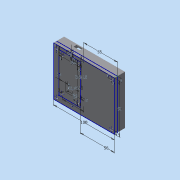
# Autodesk Inventor part: Base_V1
Saved by Autodesk Inventor 2015 (Build 190159000, 159)
## iProperties
Created: 2014-12-24
Part Number: Base_V1
Material: Generic
Document SubType Name: Modeling
Designer: Openlab
Density: 1 g/cm^3
Appearance: Default
Author: Openlab
Autodesk Inventor part; units mm, degrees
ref_plane "YZ Plane" through (0, 0, 0) normal (1, 0, 0) x (0, 1, 0)
ref_plane "XZ Plane" through (0, 0, 0) normal (0, 1, 0) x (-1, 0, 0)
ref_plane "XY Plane" through (0, 0, 0) normal (0, 0, 1) x (1, 0, 0)
sketch "Sketch1" plane through (0, 0, 0) normal (0, 1, 0) x (-1, 0, 0)
  line L0 (100, 0) -> (0, 0)
  line L1 (0, 0) -> (0, -80)
  line L2 (0, -80) -> (100, -80)
  line L3 (100, -80) -> (100, 0)
  line L4 (95, -5) -> (78, -5)
  line L5 (5, -5) -> (5, -75)
  line L6 (5, -75) -> (95, -75)
  line L7 (95, -75) -> (95, -5)
  line L8 (33.5, -10) -> (23.5, -10)
  line L9 (23.5, -10) -> (23.5, -20)
  line L10 (23.5, -20) -> (33.5, -20)
  line L11 (95, -65) -> (95, -5)
  line L12 (33.5, -50) -> (23.5, -50)
  line L13 (23.5, -50) -> (23.5, -60)
  line L14 (23.5, -60) -> (33.5, -60)
  line L15 (95, -5) -> (90, -5)
  line L16 (90, -5) -> (90, -10)
  line L17 (90, -10) -> (95, -10)
  line L18 (95, -10) -> (95, -5)
  line L19 (95, -75) -> (90, -75)
  line L20 (90, -75) -> (90, -70)
  line L21 (90, -70) -> (95, -70)
  line L22 (95, -70) -> (95, -75)
  line L23 (5, -5) -> (10, -5)
  line L24 (10, -5) -> (10, -10)
  line L25 (10, -10) -> (5, -10)
  line L26 (5, -10) -> (5, -5)
  line L27 (5, -75) -> (10, -75)
  line L28 (10, -75) -> (10, -70)
  line L29 (10, -70) -> (5, -70)
  line L30 (5, -70) -> (5, -75)
  line L31 (78, -5) -> (78, -2.5)
  line L32 (78, -2.5) -> (68, -2.5)
  line L33 (68, -2.5) -> (68, -5)
  line L34 (78, -5) -> (73, -5) construction
  line L35 (95, -5) -> (78, -5)
  line L36 (73, -5) -> (68, -5) construction
  line L37 (68, -5) -> (55, -5)
  line L38 (14.5, -63) -> (14.5, -5)
  line L39 (38.5, -63) -> (14.5, -63)
  line L40 (14.5, -5) -> (5, -5)
  line L41 (33.5, -30) -> (23.5, -30)
  line L42 (23.5, -30) -> (23.5, -40)
  line L43 (23.5, -40) -> (33.5, -40)
  line L44 (35.5, -60) -> (36.6, -60)
  line L45 (36.6, -50) -> (35.5, -50)
  line L46 (33.5, -60) -> (33.5, -56.5)
  line L47 (33.5, -53.5) -> (33.5, -50)
  line L48 (38.5, -56.5) -> (38.5, -63)
  line L49 (36.6, -60) -> (36.6, -56.5)
  line L50 (36.6, -53.5) -> (36.6, -50)
  line L51 (35.5, -50) -> (35.5, -53.5)
  line L52 (35.5, -56.5) -> (35.5, -60)
  line L53 (33.5, -56.5) -> (35.5, -56.5)
  line L54 (36.6, -56.5) -> (38.5, -56.5)
  line L55 (38.5, -53.5) -> (36.6, -53.5)
  line L56 (35.5, -53.5) -> (33.5, -53.5)
  line L57 (33.5, -40) -> (33.5, -36.5)
  line L58 (33.5, -33.5) -> (33.5, -30)
  line L59 (38.5, -36.5) -> (38.5, -53.5)
  line L60 (33.5, -20) -> (33.5, -16.5)
  line L61 (33.5, -13.5) -> (33.5, -10)
  line L62 (38.5, -5) -> (38.5, -13.5)
  line L63 (38.5, -16.5) -> (38.5, -33.5)
  line L64 (35.5, -40) -> (36.6, -40)
  line L65 (36.6, -30) -> (35.5, -30)
  line L66 (38.5, -36.5) -> (36.6, -36.5)
  line L67 (35.5, -36.5) -> (33.5, -36.5)
  line L68 (38.5, -33.5) -> (36.6, -33.5)
  line L69 (35.5, -33.5) -> (33.5, -33.5)
  line L70 (35.5, -30) -> (35.5, -33.5)
  line L71 (35.5, -36.5) -> (35.5, -40)
  line L72 (36.6, -40) -> (36.6, -36.5)
  line L73 (36.6, -33.5) -> (36.6, -30)
  line L74 (35.5, -20) -> (36.6, -20)
  line L75 (36.6, -10) -> (35.5, -10)
  line L76 (33.5, -16.5) -> (35.5, -16.5)
  line L77 (36.6, -16.5) -> (38.5, -16.5)
  line L78 (33.5, -13.5) -> (35.5, -13.5)
  line L79 (36.6, -13.5) -> (38.5, -13.5)
  line L80 (35.5, -10) -> (35.5, -13.5)
  line L81 (35.5, -16.5) -> (35.5, -20)
  line L82 (36.6, -20) -> (36.6, -16.5)
  line L83 (36.6, -13.5) -> (36.6, -10)
  line L84 (33.5, -56.5) -> (33.5, -53.5)
  line L85 (38.5, -56.5) -> (38.5, -53.5)
  line L86 (38.5, -36.5) -> (38.5, -33.5)
  line L87 (33.5, -36.5) -> (33.5, -33.5)
  line L88 (33.5, -16.5) -> (33.5, -13.5)
  line L89 (38.5, -16.5) -> (38.5, -13.5)
  line L90 (14.5, -57.5) -> (23.5, -57.5)
  line L91 (14.5, -52.5) -> (23.5, -52.5)
  line L92 (14.5, -37.5) -> (23.5, -37.5)
  line L93 (14.5, -32.5) -> (23.5, -32.5)
  line L94 (14.5, -17.5) -> (23.5, -17.5)
  line L95 (14.5, -12.5) -> (23.5, -12.5)
  line L96 (35.5, -56.5) -> (35.5, -53.5)
  line L97 (36.6, -56.5) -> (36.6, -53.5)
  line L98 (35.5, -36.5) -> (35.5, -33.5)
  line L99 (36.6, -36.5) -> (36.6, -33.5)
  line L100 (35.5, -16.5) -> (35.5, -13.5)
  line L101 (36.6, -16.5) -> (36.6, -13.5)
  line L102 (40, -5) -> (40, -63)
  line L103 (68, -5) -> (43, -5)
  line L104 (40, -5) -> (38.5, -5)
  line L105 (37, -75) -> (37, -72)
  line L106 (40, -5) -> (43, -5)
  line L107 (13, -5) -> (13, -72)
  line L108 (13, -72) -> (14.5, -72)
  line L109 (10, -71) -> (10, -5)
  line L110 (14.5, -72) -> (14.5, -75)
  line L111 (2.5002, -77.5) -> (2.5002, -2.5)
  line L112 (2.5002, -2.5) -> (97.5, -2.5)
  line L113 (97.5, -2.5) -> (97.5, -77.5)
  line L114 (97.5, -77.5) -> (2.5002, -77.5)
  line L115 (40, -63) -> (43, -63)
  line L116 (43, -75) -> (43, -72)
  line L117 (43, -63) -> (43, -5)
  line L118 (43, -72) -> (37, -72)
  dimension "d1" = 5
  dimension "d2" = 5
  dimension "d3" = 5
  dimension "d4" = 5
  dimension "d10" = 10
  dimension "d11" = 10
  dimension "d32" = 10
  dimension "d33" = 10
  dimension "d36" = 70
  dimension "d55" = 5
  dimension "d56" = 5
  dimension "d57" = 5
  dimension "d58" = 5
  dimension "d59" = 5
  dimension "d60" = 5
  dimension "d61" = 5
  dimension "d62" = 5
  dimension "d185" = 2.5
  dimension "d186" = 10
  dimension "d187" = 90
  dimension "d188" = 9.5
  dimension "d195" = 3
  dimension "d196" = 10
  dimension "d197" = 80
  dimension "d198" = 10
  dimension "d199" = 10
  dimension "d200" = 10
  dimension "d201" = 10
  dimension "d234" = 1.1
  dimension "d235" = 10
  dimension "d239" = 6.5
  dimension "d240" = 2
  dimension "d241" = 1.9
  dimension "d243" = 3.5
  dimension "d244" = 1.1
  dimension "d245" = 2
  dimension "d246" = 1.9
  dimension "d247" = 3.5
  dimension "d253" = 3
  dimension "d254" = 1.1
  dimension "d255" = 10
  dimension "d258" = 2
  dimension "d259" = 2
  dimension "d260" = 3.5
  dimension "d261" = 3.5
  dimension "d262" = 1.9
  dimension "d263" = 1.9
  dimension "d264" = 17
  dimension "d265" = 3
  dimension "d266" = 1.1
  dimension "d267" = 10
  dimension "d268" = 1.9
  dimension "d269" = 3.5
  dimension "d270" = 3.5
  dimension "d273" = 5
  dimension "d274" = 2.5
  dimension "d275" = 5
  dimension "d276" = 2.5
  dimension "d277" = 5
  dimension "d278" = 2.5
  dimension "d288" = 1.5
  dimension "d297" = 9
  dimension "d298" = 58
  dimension "d299" = 1.5
  constraints: 238 end point, 61 perpendicular, 53 parallel, 24 horizontal, 17 point on line, 16 collinear, 6 vertical, 1 coincident
  measures "d1" distance between parallel lines of L2 L6
  measures "d2" distance between parallel lines of L7 L3
  measures "d3" distance between parallel lines of L1 L5
  measures "d4" distance between parallel lines of L4 L0
  measures "d10" distance of L10.end L8.start
  measures "d11" distance of L9.end L10.end
  measures "d32" distance of L14.end L12.start
  measures "d33" distance of L13.end L14.end
  measures "d36" distance of L5.start L5.end
  measures "d55" distance of L17.end L16.end
  measures "d56" distance of L16.end L15.end
  measures "d57" distance of L20.end L21.end
  measures "d58" distance of L19.end L20.end
  measures "d59" distance of L24.end L25.end
  measures "d60" distance of L23.end L24.end
  measures "d61" distance of L29.end L28.end
  measures "d62" distance of L28.end L27.end
  measures "d185" distance of L4.end L31.end
  measures "d186" distance of L31.end L32.end
  measures "d187" distance of L5.end L6.end
  measures "d188" distance between parallel lines of L5 L38
  measures "d195" distance between parallel lines of L39 L14
  measures "d196" distance between parallel lines of L0 L8
  measures "d197" distance between parallel lines of L0 L2
  measures "d198" distance of L43.end L41.start
  measures "d199" distance of L43.start L43.end
  measures "d200" distance between parallel lines of L41 L10
  measures "d201" distance between parallel lines of L12 L43
  measures "d234" distance of L45.start L45.end
  measures "d235" distance of L44.end L45.start
  measures "d239" distance of L48.start L39.start
  measures "d240" distance of L46.end L52.start
  measures "d241" distance of L49.end L48.start
  measures "d243" distance of L52.start L44.start
  measures "d244" distance of L44.start L44.end
  measures "d245" distance of L51.end L47.start
  measures "d246" distance of L55.start L50.start
  measures "d247" distance of L45.end L51.end
  measures "d253" distance between parallel lines of L56 L53
  measures "d254" distance of L65.end L65.start
  measures "d255" distance of L65.start L64.end
  measures "d258" distance of L67.start L57.end
  measures "d259" distance of L69.start L58.start
  measures "d260" distance of L67.start L64.start
  measures "d261" distance of L65.end L69.start
  measures "d262" distance of L59.start L66.end
  measures "d263" distance of L63.end L68.end
  measures "d264" distance of L59.start L55.start
  measures "d265" distance between parallel lines of L68 L66
  measures "d266" distance of L75.end L75.start
  measures "d267" distance of L75.start L74.end
  measures "d268" distance of L77.start L63.start
  measures "d269" distance of L76.end L74.start
  measures "d270" distance of L75.end L78.end
  measures "d273" distance between parallel lines of L95 L94
  measures "d274" distance between parallel lines of L8 L95
  measures "d275" distance between parallel lines of L93 L92
  measures "d276" distance between parallel lines of L41 L93
  measures "d277" distance between parallel lines of L90 L91
  measures "d278" distance between parallel lines of L12 L91
  measures "d288" distance between parallel lines of L102 L62
  measures "d297" distance between parallel lines of L13 L38
  measures "d298" distance of L38.start L38.end
  measures "d299" distance between parallel lines of L38 L107
extrude "Extrusion1" add sketch "Sketch1" against normal blind 5 contours L3 L2 L1 L0 | L7 L17 L16 L4 | L4 L31 L112 L113 L114 L111 L33 L37 L103 L106 L104 L62 L79 L83 L75 L80 L78 L61 L8 L9 L95 L38 L40 L23 L5 L6 L7 | L16 L17 L7 L21 L20 L6 L116 L118 L105 L110 L108 L107 L40 L38 L39 L48 L85 L59 L86 L63 L89 L62 L104 L102 L115 L117 L103 L37 L33 L32 L31 L4 | L7 L6 L20 L21 | L6 L105 L118 L116 | L117 L115 L102 L106 | L6 L28 L109 L24 L40 L107 L108 L110 | L6 L5 L29 L28 | L89 L77 L101 L79 | L101 L82 L74 L81 L100 L80 L75 L83 | L63 L68 L73 L65 L70 L69 L58 L41 L42 L93 L38 L94 L9 L10 L60 L76 L81 L74 L82 L77 | L5 L25 L109 L29 | L86 L66 L99 L68 | L5 L23 L24 L25 | L99 L72 L64 L71 L98 L70 L65 L73 | L59 L55 L50 L45 L51 L56 L47 L12 L13 L91 L38 L92 L42 L43 L57 L67 L71 L64 L72 L66 | L95 L9 L94 L38 | L100 L76 L88 L78 | L85 L54 L97 L55 | L9 L8 L61 L88 L60 L10 | L97 L49 L44 L52 L96 L51 L45 L50 | L48 L39 L38 L90 L13 L14 L46 L53 L52 L44 L49 L54 | L93 L42 L92 L38 | L98 L67 L87 L69 | L42 L41 L58 L87 L57 L43 | L91 L13 L90 L38 | L96 L53 L84 L56 | L13 L12 L47 L84 L46 L14
sketch "Sketch3" plane through (0, 0, 0) normal (0, 1, 0) x (-1, 0, 0)
  line L0 (55, -5) -> (55, -70)
  line L1 (90, -70) -> (90, -5)
  line L2 (90, -5) -> (55, -5)
  line L3 (55, -70) -> (90, -70)
  line L4 (82.271, -5) -> (63.729, -5)
  line L5 (63.729, -5) -> (63.729, -48.18)
  line L6 (63.729, -48.18) -> (82.271, -48.18)
  line L7 (82.271, -48.18) -> (82.271, -5)
  line L8 (73, 1.7089) -> (73, -57.768) construction
  line L9 (77, -10) -> (69, -10)
  line L10 (69, -10) -> (69, -5)
  line L11 (69, -5) -> (77, -5)
  line L12 (77, -5) -> (77, -10)
  circle A0 centre (86, -65) radius 2.5
  circle A1 centre (60, -65) radius 2.5
  circle A2 centre (86, -10) radius 2.5
  circle A3 centre (60, -10) radius 2.5
  point P0 (0, 0)
  dimension "d37" = 35
  dimension "d38" = 65
  dimension "d39" = 5
  dimension "d40" = 4
  dimension "d41" = 5
  dimension "d42" = 5
  dimension "d43" = 18.542
  dimension "d44" = 43.18
  dimension "d45" = 8
  dimension "d46" = 5
  dimension "d47" = 55
  dimension "d48" = 5
  dimension "d119" = 18
  dimension "d148" = 5
  dimension "d149" = 5
  dimension "d150" = 5
  dimension "d151" = 5
  constraints: 26 end point, 6 parallel, 5 coincident, 4 centre point, 4 horizontal alignment, 3 horizontal, 3 perpendicular, 2 vertical alignment, 1 vertical, 2 other
  measures "d37" distance of L1.start L0.end
  measures "d38" distance of L1.end L1.start
  measures "d39" distance from line of L2 point (86, -10)
  measures "d40" distance from line of L1 point (86, -65)
  measures "d41" distance from line of L3 point (86, -65)
  measures "d42" distance from line of L0 point (60, -10)
  measures "d43" distance of L5.end L6.end
  measures "d44" distance of L4.end L5.end
  measures "d45" distance of L9.start L9.end
  measures "d46" distance of L11.end L9.start
  measures "d47" distance from line of point (0, 0) L0
  measures "d48" vertical distance of point (0, 0) point (55, -5)
  measures "d119" distance between parallel lines of L8 L0
  measures "d148" diameter of A0
  measures "d149" diameter of A1
  measures "d150" diameter of A2
  measures "d151" diameter of A3
extrude "Extrusion4" add sketch "Sketch3" along normal blind 2 contours A0 | A1 | A2 | A3
hole "Hole13" at (-86, 0, -65) direction (0, 1, 0) diameter 3 end through all
hole "Hole14" at (-86, 0, -10) direction (0, 1, 0) diameter 3 end through all
hole "Hole15" at (-60, 0, -10) direction (0, 1, 0) diameter 3 end through all
hole "Hole16" at (-60, 0, -65) direction (0, 1, 0) diameter 3 end through all
extrude "Extrusion9" add sketch "Sketch1" along normal blind 5 contours L89 L77 L101 L79 | L86 L66 L99 L68 | L95 L9 L94 L38 | L100 L76 L88 L78 | L85 L54 L97 L55 | L93 L42 L92 L38 | L98 L67 L87 L69 | L91 L13 L90 L38 | L96 L53 L84 L56
extrude "Extrusion10" add sketch "Sketch1" along normal blind 2.5 contours L101 L82 L74 L81 L100 L80 L75 L83 | L99 L72 L64 L71 L98 L70 L65 L73 | L97 L49 L44 L52 L96 L51 L45 L50
extrude "Extrusion11" add sketch "Sketch1" along normal blind 2.5 contours L6 L105 L118 L116 | L117 L115 L102 L106 | L6 L28 L109 L24 L40 L107 L108 L110 | L6 L5 L29 L28 | L5 L25 L109 L29 | L5 L23 L24 L25
sketch "Sketch5" plane through (0, -5, 0) normal (0, -1, 0) x (1, 0, 0)
  line L0 (-100, 0) -> (0, 0)
  line L1 (0, 0) -> (0, -80)
  line L2 (0, -80) -> (-100, -80)
  line L3 (-100, -80) -> (-100, 0)
  line L4 (-56, -5) -> (-56, -70)
  line L5 (-91, -70) -> (-91, -5)
  line L6 (-56, -70) -> (-91, -70)
  line L7 (-91, -5) -> (-56, -5)
  point P0 (-95, -75)
  point P1 (-95, -5)
  point P2 (-5, -5)
  point P3 (-5, -75)
  point P4 (-60, -10)
  point P5 (-86, -10)
  point P6 (-86, -65)
  point P7 (-60, -65)
  dimension "d310" = 100
  dimension "d311" = 80
  dimension "d314" = 5
  dimension "d315" = 5
  dimension "d316" = 5
  dimension "d317" = 5
  dimension "d326" = 65
  dimension "d342" = 35
  dimension "d347" = 5
  dimension "d352" = 4
  dimension "d353" = 5
  dimension "d354" = 5
  dimension "d355" = 56
  dimension "d356" = 5
  constraints: 16 end point, 4 horizontal alignment, 4 parallel, 4 vertical alignment, 2 coincident, 2 perpendicular, 1 horizontal
  measures "d310" distance of L1.end L2.end
  measures "d311" distance of L0.end L1.end
  measures "d314" distance from line of L0 point (-5, -5)
  measures "d315" distance from line of L1 point (-5, -5)
  measures "d316" distance from line of L2 point (-5, -75)
  measures "d317" distance from line of L3 point (-95, -5)
  measures "d326" distance of L4.end L4.start
  measures "d342" distance of L5.end L4.start
  measures "d347" distance from line of L5 point (-86, -10)
  measures "d352" distance from line of L4 point (-60, -10)
  measures "d353" distance from line of L7 point (-60, -10)
  measures "d354" distance from line of L6 point (-60, -65)
  measures "d355" distance between parallel lines of L1 L4
  measures "d356" distance between parallel lines of L0 L7
hole "Hole22" at (-60, -5, -10) at (-86, -5, -10) at (-86, -5, -65) at (-60, -5, -65) direction (0, 1, 0) diameter 3 end through all counterbore diameter 5 counterbore depth 2
extrude "Extrusion16" add sketch "Sketch1" along normal blind 12.5
sketch "Sketch7" plane through (-100, -5, 0) normal (0, 0, 1) x (1, 0, 0)
  line L0 (22, 16) -> (32, 16)
  line L1 (32, 16) -> (32, 11)
  line L2 (32, 11) -> (22, 11)
  line L3 (22, 11) -> (22, 16)
  line L4 (0, 17.5) -> (0, 0) projected
  point P0 (100, 5)
  dimension "d380" = 10
  dimension "d381" = 5
  dimension "d382" = 22
  dimension "d383" = 11
  constraints: 8 end point, 2 parallel, 1 horizontal, 1 perpendicular
  measures "d380" distance of L1.end L2.end
  measures "d381" distance of L0.end L1.end
  measures "d382" distance between parallel lines of L4 L3
  measures "d383" distance from line of L4.end L2
extrude "Extrusion17" cut sketch "Sketch7" against normal blind 12.5
extrude "Extrusion18" add sketch "Sketch1" along normal blind 15 contours L7 L17 L16 L4 | L4 L31 L112 L113 L114 L111 L33 L37 L103 L106 L104 L62 L79 L83 L75 L80 L78 L61 L8 L9 L95 L38 L40 L23 L5 L6 L7 | L7 L6 L20 L21 | L6 L5 L29 L28 | L63 L68 L73 L65 L70 L69 L58 L41 L42 L93 L38 L94 L9 L10 L60 L76 L81 L74 L82 L77 | L5 L23 L24 L25 | L59 L55 L50 L45 L51 L56 L47 L12 L13 L91 L38 L92 L42 L43 L57 L67 L71 L64 L72 L66 | L48 L39 L38 L90 L13 L14 L46 L53 L52 L44 L49 L54
hole "Hole21" at (-5, -5, -5) at (-95, -5, -5) at (-95, -5, -75) at (-5, -5, -75) direction (0, 1, 0) diameter 3 depth 20 tip angle 118 counterbore diameter 5 counterbore depth 2
fillet "Fillet3" radius 2.5 6 edges at (-19, 5, -57.5) (-19, 5, -52.5) (-19, 5, -37.5) (-19, 5, -32.5) (-19, 5, -17.5) (-19, 5, -12.5)
body "Solid1"
